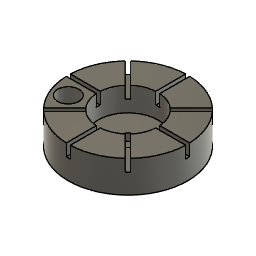
Reifenhalterung v2 (Autodesk Fusion 360 archive; units mm, degrees)
design "Reifenhalterung" references "Sechskantmutter JIS B 1181 - M8 - Klasse 1 halb-bearbeitet Stahl 6 Einfach"
Autodesk Fusion 360 part; units mm, degrees
note: some values were not read from the file. Chosen so that the rebuilt part matches the saved one: which sketch regions a step uses; how an offset face is resized.
sketch "Skizze1" plane through (0, 0, 0) normal (0, 1, 0) x (1, 0, 0)
  circle A0 centre (0, 0) radius 60
  dimension "d1" = 120
  constraint coincident A0.centre origin
  measures "d1" diameter of A0
extrude "Extrusion1" add sketch "Skizze1" along normal blind 5 makes body 1
sketch "Skizze2" plane through (0, 0, 0) normal (0, 1, 0) x (1, 0, 0)
  circle A0 centre (150, 0) radius 60
  circle A1 centre (150, 0) radius 45
  line L0 (150, 0) -> (150, 1.5)
  line L1 (150, 0) -> (150, -1.5)
  line L2 (150, -1.5) -> (105.025, -1.5)
  line L3 (150, 1.5) -> (105.025, 1.5)
  line L4 (150, 0) -> (151.5, 0)
  line L5 (151.5, 0) -> (151.5, 44.975)
  line L6 (150, 0) -> (148.5, 0)
  line L7 (148.5, 0) -> (148.5, 44.975)
  line L8 (150, 1.5) -> (209.9812, 1.5)
  line L9 (150, -1.5) -> (209.9812, -1.5)
  line L10 (148.5, 0) -> (148.5, -44.975)
  line L11 (151.5, -1.5) -> (151.5, -44.975)
  line L12 (150, 0) -> (150.5, 0.5)
  line L13 (150.5, 0.5) -> (149.4393, 1.5607)
  line L14 (150.5, 0.5) -> (151.5607, -0.5607)
  line L15 (151.5607, -0.5607) -> (182.8627, 30.7416)
  line L16 (149.4393, 1.5607) -> (180.7414, 32.8629)
  line L17 (151.5607, -0.5607) -> (119.2586, -32.8629)
  line L18 (149.4393, 1.5607) -> (117.1373, -30.7416)
  line L19 (150, 0) -> (146.0023, 3.9977)
  line L20 (146.0023, 3.9977) -> (147.063, 5.0583)
  line L21 (146.0023, 3.9977) -> (144.9417, 2.937)
  line L22 (147.063, 5.0583) -> (119.2584, 32.8627)
  line L23 (144.9417, 2.937) -> (117.1371, 30.7414)
  line L24 (144.9417, 2.937) -> (180.7416, -32.8627)
  line L25 (147.063, 5.0583) -> (182.8629, -30.7414)
  circle A2 centre (150, 0) radius 22.5
  dimension "d6" = 1.5
  dimension "d7" = 1.5
  dimension "d8" = 1.5
  dimension "d9" = 1.5
  dimension "d10" = 1.5
  dimension "d11" = 1.5
  dimension "d12" = 45
  constraint concentric A0 A1
  constraint coincident A0.centre A1.centre
  constraint vertical L0
  constraint parallel L0 L1
  constraint coincident A1 L2.end
  constraint perpendicular L1 L2
  constraint coincident A1 L3.end
  constraint perpendicular L0 L3
  constraint perpendicular L0 L4
  constraint coincident A1 L5.end
  constraint perpendicular L4 L5
  constraint perpendicular L1 L6
  constraint coincident A1 L7.end
  constraint perpendicular L3 L7
  constraint coincident A0 L8.end
  constraint perpendicular L1 L8
  constraint coincident A0 L9.end
  constraint perpendicular L1 L9
  constraint coincident A1 L10.end
  constraint perpendicular L2 L10
  constraint coincident L9 L11.start
  constraint coincident A1 L11.end
  constraint perpendicular L9 L11
  constraint perpendicular L12 L13
  constraint perpendicular L12 L14
  constraint coincident A1 L15.end
  constraint perpendicular L14 L15
  constraint coincident A1 L16.end
  constraint perpendicular L13 L16
  constraint coincident A1 L17.end
  constraint perpendicular L14 L17
  constraint coincident A1 L18.end
  constraint perpendicular L13 L18
  constraint perpendicular L12 L19
  constraint perpendicular L19 L20
  constraint perpendicular L19 L21
  constraint coincident A1 L22.end
  constraint perpendicular L20 L22
  constraint coincident A1 L23.end
  constraint perpendicular L21 L23
  constraint coincident A1 L24.end
  constraint perpendicular L17 L24
  constraint coincident A1 L25.end
  constraint perpendicular L16 L25
  constraint concentric A0 A2
  measures "d6" distance of A0.centre L0.end
  measures "d7" distance of A0.centre L1.end
  measures "d8" distance of L12.end L13.end
  measures "d9" distance of L12.end L14.end
  measures "d10" distance of L19.end L20.end
  measures "d11" distance of L19.end L21.end
  measures "d12" diameter of A2
extrude "Extrusion2" add sketch "Skizze2" along normal blind 15 separate body contours A1 L8 L15 A2 | A1 L9 L25 A2 | A1 L5 L16 A2 | A1 L11 L24 A2 | A1 L7 L22 A2 | A1 L10 L17 A2 | A1 L3 L23 A2 | A1 L2 L18 A2 makes body 2 at (173.7575, 0, 28.9084) makes body 3 at (126.2425, 0, -28.9084) makes body 4 at (173.7573, 0, -28.9086) makes body 5 at (126.2427, 0, 28.9086) makes body 6 at (187.2404, 0, 3.6424) makes body 7 at (112.7596, 0, -3.6424) makes body 8 at (178.9084, 0, -23.7575) makes body 9 at (112.7596, 0, 3.6424)
extrude "Extrusion3" cut 8 faces at (112.7596, 15, -3.6424) (126.2425, 15, -28.9084) (173.7573, 15, -28.9086) (178.9084, 15, -23.7575) (187.2404, 15, 3.6424) (173.7575, 15, 28.9084) (126.2427, 15, 28.9086) (112.7596, 15, 3.6424) along direction (0, -1, 0) blind 6 on bodies 2 3 4 5 6 7 8 9 bodies 2 3 4 5 6 7 8 9
extrude "Extrusion4" add 1 faces at (15.3262, 5, -22.4794) along direction (0, 1, 0) blind 20 on bodies 1 bodies 1
hole "Bohrung1" at (0, 25, 0) direction (0, -1, 0) diameter 8.036 depth 60 tip angle 180 bodies 1
thread "Gewinde1" "ISO Metric profile 9.0 M9x1 6H" thread offset 0 thread depth 7.4
sketch "Skizze3" plane through (0, 0, 0) normal (0, 1, 0) x (1, 0, 0)
hole "Bohrung2" at (0, 25, 0) direction (0, -1, 0) diameter 45 depth 9 tip angle 180 bodies 1
sketch "Skizze4" plane through (0, 0, 0) normal (0, 1, 0) x (1, 0, 0)
  circle A0 centre (-175, 0) radius 60
  circle A1 centre (-175, 0) radius 45
  dimension "d27" = 120
  dimension "d28" = 90
  constraint concentric A0 A1
  measures "d27" diameter of A0
  measures "d28" diameter of A1
extrude "Extrusion5" add sketch "Skizze4" along normal blind 3 separate body makes body 10
move_body "Verschieben1" bodies 10 to x (1, 0, 0) y (0, 1, 0) z (0, 0, 1) at (175, 60, 0)
extrude "Extrusion6" add 1 faces at (54.7766, 60, 2.9808) along direction (0, -1, 0) blind 90 on bodies 10 bodies 1 10
extrude "Extrusion7" cut 1 faces at (54.7766, 63, 2.9808) along direction (0, -1, 0) blind 120 on bodies 1 bodies 1
sketch "Skizze5" plane through (0, 0, 0) normal (0, 1, 0) x (1, 0, 0)
other "Mutter1"
sketch "Skizze6" plane through (0, 0, 0) normal (0, 1, 0) x (1, 0, 0)
extrude "Extrusion8" cut 1 faces at (31.1681, 0, 2.3357) along direction (0, 1, 0) blind 5 on bodies 1 bodies 1
extrude "Extrusion9" cut 1 faces at (31.1681, 5, 2.3357) along direction (0, 1, 0) blind 5 on bodies 1 bodies 1
move_body "Verschieben2" bodies 9 7 5 4 2 3 6 8 to x (1, 0, 0) y (0, 1, 0) z (0, 0, 1) at (-150, 25, 0)
hole "Bohrung3" at (-31.8237, 34, 13.1819) direction (0, -1, 0) diameter 16 depth 51 tip angle 180 bodies 1 9
copy_body "Körper kopieren/einfügen1" bodies 2 1 3 4 5 6 7 8 9 makes body 11 makes body 12 makes body 13 makes body 14 makes body 15 makes body 16 makes body 17 makes body 18 makes body 19
move_body "Verschieben3" bodies 11 12 13 14 15 16 17 18 19 to x (1, 0, 0) y (0, 1, 0) z (0, 0, 1) at (-120, 0, 0)
combine "Kombinieren1" operation add target body 2 tool bodies 1 5 8 3 7 4 9 6
move_body "Verschieben4" bodies 2 to x (1, 0, 0) y (0, 1, 0) z (0, 0, 1) at (0, -10, 0)
component "Reifenhalterung v2" placed x (1, 0, 0) y (0, 1, 0) z (0, 0, 1) at (0, 0, 0)
hidden bodies 11 12 13 14 15 16 17 18 19

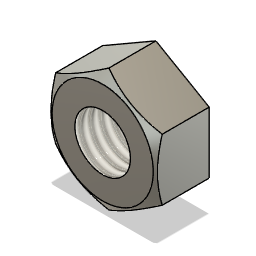
design "Sechskantmutter JIS B 1181 - M8 - Klasse 1 halb-bearbeitet Stahl 6 Einfach"
description: Sechskantmutter JIS B 1181 - M8 - Klasse 1 halb-bearbeitet
Autodesk Fusion 360 part; units mm, degrees
sketch "Sketch1" plane through (0, 0, 0) normal (0, 1, 0) x (1, 0, 0)
  line L0 (0, 0) -> (0, -6.5)
  line L1 (-7.5075, 0) -> (-7.5075, -5.7307)
  line L2 (-7.5075, -5.7307) -> (-6.175, -6.5)
  line L3 (-7.5075, 0) -> (-4, 0)
  line L4 (-4, 0) -> (-4, -6.5)
  line L5 (-4, -6.5) -> (-6.175, -6.5)
  dimension "d81" = 15.015
  dimension "d121" = 6.5
  dimension "d122" = 8
  dimension "d123" = 30
  dimension "d124" = 12.35
  dimension "d133" = 6.5
  constraint vertical L0
  constraint parallel L0 L1
  constraint coincident L0 L0.end
  constraint coincident origin L0
  constraint perpendicular L1 L3
  constraint perpendicular L3 L4
  constraint perpendicular L4 L5
  constraint coincident L0.start L3
  constraint coincident L0.start origin
  measures "d121" distance of L3.end L4.end
  measures "d123" angle of L2 L5
  measures "d133" distance of L0.start L0.end
revolve "Revolve1" add sketch "Sketch1" angle 360 about axis through (0, 0, 0) along (0, 0, 1)
sketch "Sketch8" plane through (0, 0, 6.5) normal (0, 0, 1) x (1, 0, 0)
  line L0 (0, 0) -> (-13, 0) construction
  line L1 (-6.5, -3.7567) -> (-6.5, 3.7567)
  circle A0 centre (0, 0) radius 7.5075
  dimension "d114" = 6.5
  constraint horizontal L0
  constraint perpendicular L0 L1
  constraint midpoint L0 L1
  constraint coincident L0.start A0.centre
  constraint coincident L1.end A0
  measures "d114" distance of L0.start L1
extrude "Extrude5" cut sketch "Sketch8" against normal blind 6.5 contours L1 A0 picked at (-6.6626, -0.915)
pattern_circular "C-Pattern2" count 6 over 360 about axis through (0, 0, 1.75) along (0, 0, 1) of "Extrude5"
thread "Thread3" "ISO Metric profile 8.0 M8x1.25 6H" major diameter 8.17 minor diameter 6.7795 pitch 1.25 angle 60 resizes the face on face at (-3.9801, 0.3983, 4.3333)
equation "adsk_nheig = 6.50 mm"
equation "adsk_maxdia = 15.015 mm"
equation "adsk_nomdia = 8.00 mm"
equation "d81 = adsk_maxdia"
equation "d89 = -adsk_nheig"
equation "adsk_waflat = 13.00 mm"
equation "d114 = adsk_waflat / 2"
equation "adsk_chamang2 = 30.00 deg"
equation "d121 = adsk_nheig"
equation "d122 = adsk_nomdia"
equation "d123 = adsk_chamang2"
equation "d124 = adsk_waflat * 0.95"
equation "d131 = adsk_nheig"
equation "d133 = adsk_nheig"
